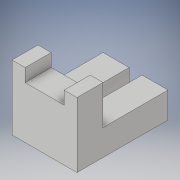
# Autodesk Inventor part: Part1
Saved by Autodesk Inventor 2017 (Build 210142000, 142)
## iProperties
Created: 2016-11-01
Part Number: Part1
Material: Generic
Document SubType Name: Modeling
Designer: s411888
Density: 1 g/cm^3
Appearance: Default
Author: s411888
Autodesk Inventor part; units mm, degrees
ref_plane "YZ Plane" through (0, 0, 0) normal (1, 0, 0) x (0, 1, 0)
ref_plane "XZ Plane" through (0, 0, 0) normal (0, 1, 0) x (-1, 0, 0)
ref_plane "XY Plane" through (0, 0, 0) normal (0, 0, 1) x (1, 0, 0)
sketch "Sketch1" plane through (0, 0, 0) normal (1, 0, 0) x (0, 1, 0)
  line L0 (8.0309, 4.2108) -> (-23.7191, 4.2108)
  line L1 (-23.7191, 4.2108) -> (-23.7191, -8.4892)
  line L2 (-23.7191, -8.4892) -> (8.0309, -8.4892)
  line L3 (8.0309, -8.4892) -> (8.0309, 4.2108)
  line L4 (-23.7191, 4.2108) -> (-11.0191, 4.2108)
  line L5 (-11.0191, 4.2108) -> (-11.0191, -40.2392)
  line L6 (-11.0191, -40.2392) -> (-23.7191, -40.2392)
  line L7 (-23.7191, -40.2392) -> (-23.7191, 4.2108)
  point P0 (0, 0)
  dimension "d0" = 31.75
  dimension "d1" = 12.7
  dimension "d2" = 44.45
  dimension "d3" = 12.7
  constraints: 16 end point, 4 parallel, 2 horizontal, 2 perpendicular
  measures "d0" distance of L2.end L1.end
  measures "d1" distance of L5.end L6.end
  measures "d2" distance of L4.end L5.end
  measures "d3" distance of L2.end L0.start
extrude "Extrusion1" add sketch "Sketch1" along normal blind 31.75
sketch "Sketch2" plane through (0, -11.0191, -8.4892) normal (0, 1, 0) x (1, 0, 0)
  line L0 (0, 31.75) -> (31.75, 31.75) projected
  line L1 (12.7448, 31.75) -> (19.0948, 31.75)
  line L2 (19.0948, 31.75) -> (19.0948, 12.7)
  line L3 (19.0948, 12.7) -> (12.7448, 12.7)
  line L4 (12.7448, 12.7) -> (12.7448, 31.75)
  line L5 (0, -12.7) -> (0, 31.75) projected
  line L6 (0, 31.75) -> (12.7, 31.75)
  line L7 (12.7, 31.75) -> (12.7, 29.079)
  line L8 (0, 29.079) -> (0, 31.75)
  point P0 (0, -8.4892)
  dimension "d6" = 6.35
  dimension "d7" = 19.05
  dimension "d8" = 12.7
  constraints: 14 end point, 3 parallel, 2 horizontal, 2 perpendicular, 1 point on line
  measures "d6" distance of L2.end L3.end
  measures "d7" distance of L1.end L2.end
  measures "d8" distance of L7.end L8.start
extrude "Extrusion2" cut sketch "Sketch2" against normal blind 12.7
sketch "Sketch3" plane through (0, 8.0309, 4.2108) normal (0, 1, 0) x (1, 0, 0)
  line L0 (0, 0) -> (31.75, 0) projected
  line L1 (31.75, 0) -> (25.4697, 0)
  line L2 (25.4697, 0) -> (25.4697, 6.35)
  line L3 (25.4697, 0) -> (6.4197, 0)
  line L4 (6.4197, 0) -> (6.4197, 12.7)
  line L5 (6.4197, 12.7) -> (25.4697, 12.7)
  line L6 (25.4697, 12.7) -> (25.4697, 0)
  line L7 (0, 0) -> (6.35, 0)
  line L8 (6.35, 0) -> (6.35, 2.265)
  line L9 (0, 2.265) -> (0, 0)
  point P0 (0, 4.2108)
  dimension "d11" = 6.35
  dimension "d12" = 19.05
  dimension "d13" = 12.7
  constraints: 18 end point, 3 horizontal, 3 parallel, 3 perpendicular
  measures "d11" distance of L1.end L2.end
  measures "d12" distance of L4.end L5.end
  measures "d13" distance of L3.end L4.end
extrude "Extrusion3" cut sketch "Sketch3" against normal blind 6.35
body "Solid1"
